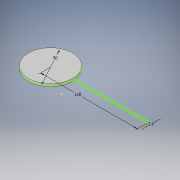
# Autodesk Inventor part: Kreisverkehrsschild_Teil_Oben
Saved by Autodesk Inventor 2019.5 (Build 235369000, 369)
## iProperties
Created: 2021-09-30
Part Number: Kreisverkehrsschild_Teil_Oben
Material: Generisch
Document SubType Name: Modeling
Designer: mritt
Density: 1 g/cm^3
Appearance: Vorgabe
Author: mritt
Autodesk Inventor part; units mm, degrees
ref_plane "YZ Plane" through (0, 0, 0) normal (1, 0, 0) x (0, 1, 0)
ref_plane "XZ Plane" through (0, 0, 0) normal (0, 1, 0) x (-1, 0, 0)
ref_plane "XY Plane" through (0, 0, 0) normal (0, 0, 1) x (1, 0, 0)
sketch "Skizze1" plane through (0, 0, 0) normal (0, 1, 0) x (-1, 0, 0)
  circle A0 centre (32.7504, -19.9257) radius 25
  line L0 (32.7504, -19.9257) -> (-77.2496, -19.9257)
  line L1 (-77.2496, -19.9257) -> (-77.2496, -22.4257)
  line L2 (-77.2496, -22.4257) -> (7.8757, -22.4257)
  line L3 (7.8757, -22.4257) -> (7.8757, -19.9257)
  point P0 (0, 0)
  dimension "d4" = 50
  dimension "d9" = 110
  dimension "d10" = 2.5
  constraints: 8 end point, 2 horizontal, 1 perpendicular, 1 point on line, 1 vertical, 3 other
  measures "d9" distance of L0.start L0.end
  measures "d10" distance of L0.end L1.end
extrude "Extrusion1" add sketch "Skizze1" along normal blind 1.5 and the other way blind 1.5 contours L3 L0 A0 | A0 L0 L3
